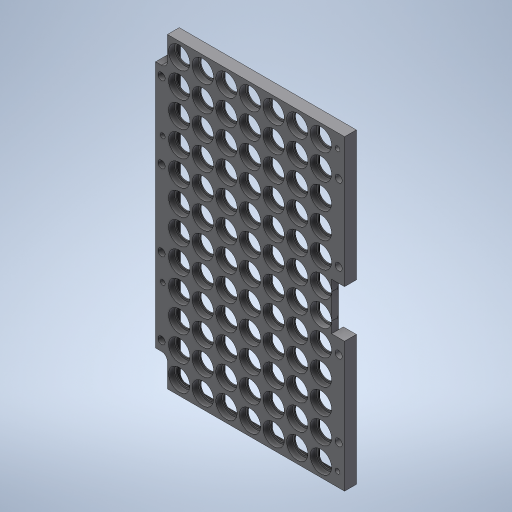
# Autodesk Inventor part: Platte2
Saved by Autodesk Inventor 2024 (Build 280153000, 153)
## iProperties
Created: 2025-03-19
Part Number: Platte2
Material: Generisch
Document SubType Name: Modeling
Designer: David Lill
Density: 1 g/cm^3
Appearance: Vorgabe
Author: David Lill
Autodesk Inventor part; units mm, degrees
ref_plane "YZ Plane" through (0, 0, 0) normal (1, 0, 0) x (0, 1, 0)
ref_plane "XZ Plane" through (0, 0, 0) normal (0, 1, 0) x (-1, 0, 0)
ref_plane "XY Plane" through (0, 0, 0) normal (0, 0, 1) x (1, 0, 0)
sketch "Skizze1" plane through (0, 0, 0) normal (0, 1, 0) x (-1, 0, 0)
  line L0 (160, 0) -> (0, 0)
  line L1 (0, 0) -> (0, -260)
  line L2 (0, -260) -> (160, -260)
  line L3 (160, -260) -> (160, 0)
  circle A0 centre (140, -11.75) radius 9
  circle A1 centre (140, -54.75) radius 9
  circle A2 centre (140, -97.75) radius 9
  circle A3 centre (140, -140.75) radius 9
  circle A4 centre (140, -183.75) radius 9
  circle A5 centre (140, -226.75) radius 9
  circle A6 centre (120, -11.75) radius 9
  circle A7 centre (120, -54.75) radius 9
  circle A8 centre (120, -97.75) radius 9
  circle A9 centre (120, -140.75) radius 9
  circle A10 centre (120, -183.75) radius 9
  circle A11 centre (120, -226.75) radius 9
  circle A12 centre (100, -11.75) radius 9
  circle A13 centre (100, -54.75) radius 9
  circle A14 centre (100, -97.75) radius 9
  circle A15 centre (100, -140.75) radius 9
  circle A16 centre (100, -183.75) radius 9
  circle A17 centre (100, -226.75) radius 9
  circle A18 centre (80, -11.75) radius 9
  circle A19 centre (80, -54.75) radius 9
  circle A20 centre (80, -97.75) radius 9
  circle A21 centre (80, -140.75) radius 9
  circle A22 centre (80, -183.75) radius 9
  circle A23 centre (80, -226.75) radius 9
  circle A24 centre (60, -11.75) radius 9
  circle A25 centre (60, -54.75) radius 9
  circle A26 centre (60, -97.75) radius 9
  circle A27 centre (60, -140.75) radius 9
  circle A28 centre (60, -183.75) radius 9
  circle A29 centre (60, -226.75) radius 9
  circle A30 centre (40, -11.75) radius 9
  circle A31 centre (40, -54.75) radius 9
  circle A32 centre (40, -97.75) radius 9
  circle A33 centre (40, -140.75) radius 9
  circle A34 centre (40, -183.75) radius 9
  circle A35 centre (40, -226.75) radius 9
  circle A36 centre (20, -11.75) radius 9
  circle A37 centre (20, -54.75) radius 9
  circle A38 centre (20, -97.75) radius 9
  circle A39 centre (20, -140.75) radius 9
  circle A40 centre (20, -183.75) radius 9
  circle A41 centre (20, -226.75) radius 9
  circle A42 centre (140, -33.25) radius 9
  circle A43 centre (120, -33.25) radius 9
  circle A44 centre (100, -33.25) radius 9
  circle A45 centre (80, -33.25) radius 9
  circle A46 centre (60, -33.25) radius 9
  circle A47 centre (40, -33.25) radius 9
  circle A48 centre (20, -33.25) radius 9
  circle A49 centre (140, -76.25) radius 9
  circle A50 centre (120, -76.25) radius 9
  circle A51 centre (100, -76.25) radius 9
  circle A52 centre (80, -76.25) radius 9
  circle A53 centre (60, -76.25) radius 9
  circle A54 centre (40, -76.25) radius 9
  circle A55 centre (20, -76.25) radius 9
  circle A56 centre (140, -119.25) radius 9
  circle A57 centre (120, -119.25) radius 9
  circle A58 centre (100, -119.25) radius 9
  circle A59 centre (80, -119.25) radius 9
  circle A60 centre (60, -119.25) radius 9
  circle A61 centre (40, -119.25) radius 9
  circle A62 centre (20, -119.25) radius 9
  circle A63 centre (140, -162.25) radius 9
  circle A64 centre (120, -162.25) radius 9
  circle A65 centre (100, -162.25) radius 9
  circle A66 centre (80, -162.25) radius 9
  circle A67 centre (60, -162.25) radius 9
  circle A68 centre (40, -162.25) radius 9
  circle A69 centre (20, -162.25) radius 9
  circle A70 centre (140, -205.25) radius 9
  circle A71 centre (120, -205.25) radius 9
  circle A72 centre (100, -205.25) radius 9
  circle A73 centre (80, -205.25) radius 9
  circle A74 centre (60, -205.25) radius 9
  circle A75 centre (40, -205.25) radius 9
  circle A76 centre (20, -205.25) radius 9
  circle A77 centre (140, -248.25) radius 9
  circle A78 centre (120, -248.25) radius 9
  circle A79 centre (100, -248.25) radius 9
  circle A80 centre (80, -248.25) radius 9
  circle A81 centre (60, -248.25) radius 9
  circle A82 centre (40, -248.25) radius 9
  circle A83 centre (20, -248.25) radius 9
  line L4 (-20, 0) -> (-187, 0)
  line L5 (-207, 0) -> (-374, 0)
  circle A84 centre (140, -11.75) radius 7.5
  line L6 (155.379, -44.5989) -> (146.379, -44.5989)
  line L7 (157, -62) -> (150, -62)
  line L8 (150, -62) -> (150, -69)
  line L9 (150, -69) -> (157, -69)
  line L10 (157, -69) -> (157, -62)
  line L11 (160, -130) -> (0, -130) construction
  line L12 (157, -198) -> (150, -198)
  line L13 (150, -198) -> (150, -191)
  line L14 (150, -191) -> (157, -191)
  line L15 (157, -191) -> (157, -198)
  point P0 (80, 0)
  point P1 (153.5, -62)
  point P2 (157, -65.5)
  dimension "d0" = 160
  dimension "d1" = 260
  dimension "d4" = 18
  dimension "d7" = 43
  dimension "d10" = 20
  dimension "d16" = 21.5
  dimension "d21" = 20
  dimension "d24" = 43
  dimension "d69" = 15
  dimension "d80" = 0
  dimension "d127" = 10.75
  dimension "d129" = 7
  dimension "d130" = 7
  dimension "d132" = 3
  dimension "d134" = 10.75
  constraints: 85 centre point, 32 end point, 14 coincident, 6 horizontal, 5 midpoint, 4 parallel, 4 symmetric about line, 2 horizontal alignment, 2 perpendicular, 2 vertical, 1 equal radius, 1 vertical alignment, 164 other
  measures "d0" distance of L0.start L0.end
  measures "d1" distance of L2.end L0.start
  measures "d4" diameter of A0
  measures "d7" distance of A0.centre A1.centre
  measures "d10" distance of A0.centre A6.centre
  measures "d16" distance of A42.centre A0.centre
  measures "d21" distance of A42.centre A43.centre
  measures "d24" distance of A42.centre A49.centre
  measures "d69" diameter of A84
  measures "d80" horizontal distance of A0.centre A42.centre
  measures "d127" vertical distance of L11.start point (140, -119.25)
  measures "d129" distance of L9.end L8.end
  measures "d130" distance of L8.end L7.end
  measures "d132" distance between parallel lines of L3 L10
  measures "d134" vertical distance of point (140, -76.25) point (157, -65.5)
extrude "Extrusion1" add sketch "Skizze1" along normal blind 10 contours L3 L2 L1 L0 | A0 | A1 | A2 | A3 | A4 | A5 | A6 | A7 | A8 | A9 | A10 | A11 | A12 | A13 | A14 | A15 | A16 | A17 | A18 | A19 | A20 | A21 | A22 | A23 | A24 | A25 | A26 | A27 | A28 | A29 | A30 | A31 | A32 | A33 | A34 | A35 | A36 | A37 | A38 | A39 | A40 | A41 | A42 | A43 | A44 | A45 | A46 | A47 | A48 | A49 | A50 | A51 | A52 | A53 | A54 | A55 | A56 | A57 | A58 | A59 | A60 | A61 | A62 | A63 | A64 | A65 | A66 | A67 | A68 | A69 | A70 | A71 | A72 | A73 | A74 | A75 | A76 | A77 | A78 | A79 | A80 | A81 | A82 | A83 | A84 | L10 L9 L8 L7 | L12 L13 L14 L15
hole "Bohrung1" at (-140, 0, -11.75) at (-140, 0, -33.25) at (-140, 0, -54.75) at (-140, 0, -76.25) at (-140, 0, -97.75) at (-140, 0, -119.25) at (-140, 0, -140.75) at (-140, 0, -162.25) at (-140, 0, -183.75) at (-140, 0, -205.25) at (-140, 0, -226.75) at (-140, 0, -248.25) direction (0, 1, 0) diameter 15 end through all counterbore diameter 18 counterbore depth 5
pattern_linear "Rechteckige Anordnung1" count 7 spacing 20 along (1, 0, 0) of "Bohrung1"
sketch "Skizze2" plane through (0, 10, 0) normal (0, 1, 0) x (1, 0, 0)
  circle A0 centre (-20, 226.75) radius 9 projected
  circle A1 centre (-20, 248.25) radius 9 projected
  circle A2 centre (-20, 205.25) radius 9 projected
  circle A3 centre (-20, 162.25) radius 9 projected
  circle A4 centre (-20, 119.25) radius 9 projected
  circle A5 centre (-20, 33.25) radius 9 projected
  circle A6 centre (-20, 11.75) radius 9
  circle A7 centre (-20, 54.75) radius 9 projected
  circle A8 centre (-20, 97.75) radius 9 projected
  circle A9 centre (-20, 140.75) radius 9 projected
  circle A10 centre (-20, 183.75) radius 9 projected
  circle A11 centre (-40, 226.75) radius 9 projected
  circle A12 centre (-40, 248.25) radius 9 projected
  circle A13 centre (-40, 205.25) radius 9 projected
  circle A14 centre (-40, 162.25) radius 9 projected
  circle A15 centre (-40, 119.25) radius 9 projected
  circle A16 centre (-40, 76.25) radius 9 projected
  circle A17 centre (-40, 33.25) radius 9 projected
  circle A18 centre (-40, 11.75) radius 9 projected
  circle A19 centre (-40, 54.75) radius 9 projected
  circle A20 centre (-40, 97.75) radius 9 projected
  circle A21 centre (-40, 140.75) radius 9 projected
  circle A22 centre (-40, 183.75) radius 9 projected
  circle A23 centre (-60, 226.75) radius 9 projected
  circle A24 centre (-60, 248.25) radius 9 projected
  circle A25 centre (-60, 205.25) radius 9 projected
  circle A26 centre (-60, 162.25) radius 9 projected
  circle A27 centre (-60, 119.25) radius 9 projected
  circle A28 centre (-60, 76.25) radius 9 projected
  circle A29 centre (-60, 33.25) radius 9 projected
  circle A30 centre (-60, 11.75) radius 9 projected
  circle A31 centre (-60, 54.75) radius 9 projected
  circle A32 centre (-60, 97.75) radius 9 projected
  circle A33 centre (-60, 140.75) radius 9 projected
  circle A34 centre (-60, 183.75) radius 9 projected
  circle A35 centre (-80, 226.75) radius 9 projected
  circle A36 centre (-80, 248.25) radius 9 projected
  circle A37 centre (-80, 205.25) radius 9 projected
  circle A38 centre (-80, 162.25) radius 9 projected
  circle A39 centre (-80, 119.25) radius 9 projected
  circle A40 centre (-80, 76.25) radius 9 projected
  circle A41 centre (-80, 33.25) radius 9 projected
  circle A42 centre (-80, 11.75) radius 9 projected
  circle A43 centre (-80, 54.75) radius 9 projected
  circle A44 centre (-80, 97.75) radius 9 projected
  circle A45 centre (-80, 140.75) radius 9 projected
  circle A46 centre (-80, 183.75) radius 9 projected
  circle A47 centre (-100, 226.75) radius 9 projected
  circle A48 centre (-100, 248.25) radius 9 projected
  circle A49 centre (-100, 205.25) radius 9 projected
  circle A50 centre (-100, 162.25) radius 9 projected
  circle A51 centre (-100, 119.25) radius 9 projected
  circle A52 centre (-100, 76.25) radius 9 projected
  circle A53 centre (-100, 33.25) radius 9 projected
  circle A54 centre (-100, 11.75) radius 9 projected
  circle A55 centre (-100, 54.75) radius 9 projected
  circle A56 centre (-100, 97.75) radius 9 projected
  circle A57 centre (-100, 140.75) radius 9 projected
  circle A58 centre (-100, 183.75) radius 9 projected
  circle A59 centre (-120, 226.75) radius 9 projected
  circle A60 centre (-120, 248.25) radius 9 projected
  circle A61 centre (-120, 205.25) radius 9 projected
  circle A62 centre (-120, 162.25) radius 9 projected
  circle A63 centre (-120, 119.25) radius 9 projected
  circle A64 centre (-120, 76.25) radius 9 projected
  circle A65 centre (-120, 33.25) radius 9 projected
  circle A66 centre (-120, 11.75) radius 9 projected
  circle A67 centre (-120, 54.75) radius 9 projected
  circle A68 centre (-120, 97.75) radius 9 projected
  circle A69 centre (-120, 140.75) radius 9 projected
  circle A70 centre (-120, 183.75) radius 9 projected
  circle A71 centre (-140, 226.75) radius 9 projected
  circle A72 centre (-140, 183.75) radius 9 projected
  circle A73 centre (-140, 140.75) radius 9 projected
  circle A74 centre (-140, 97.75) radius 9 projected
  circle A75 centre (-140, 54.75) radius 9 projected
  circle A76 centre (-140, 11.75) radius 9 projected
  circle A77 centre (-140, 33.25) radius 9 projected
  circle A78 centre (-140, 76.25) radius 9 projected
  circle A79 centre (-140, 119.25) radius 9 projected
  circle A80 centre (-140, 162.25) radius 9 projected
  circle A81 centre (-140, 205.25) radius 9 projected
  circle A82 centre (-140, 248.25) radius 9 projected
  line L0 (0, 0) -> (0, 260) projected
  line L1 (-160, 0) -> (0, 0) projected
  line L2 (-160, 260) -> (-160, 0) projected
  line L3 (0, 260) -> (-160, 260) projected
  line L4 (-160, 0) -> (0, 0) projected
  line L5 (-150, 0) -> (-150, 55)
  arc A83 (-150, 55) -> (-155, 60) centre (-155, 55) ccw
  line L6 (-155, 60) -> (-160, 60)
  line L7 (-160, 260) -> (-160, 0) projected
  line L8 (-160, 0) -> (0, 0) projected
  line L9 (0, 0) -> (0, 260) projected
  line L10 (-160, 260) -> (-160, 0) projected
  line L11 (0, 260) -> (-160, 260) projected
  line L12 (-160, 25) -> (-155, 25)
  arc A84 (-150, 20) -> (-155, 25) centre (-155, 20) ccw
  line L13 (0, 130) -> (-160, 130)
  line L14 (-150, 260) -> (-150, 205)
  arc A85 (-155, 200) -> (-150, 205) centre (-155, 205) ccw
  line L15 (-155, 200) -> (-160, 200)
  line L16 (-160, 235) -> (-155, 235)
  arc A86 (-155, 235) -> (-150, 240) centre (-155, 240) ccw
  circle A87 centre (-20, 11.75) radius 9 projected
  line L17 (-143.0414, 85.25) -> (-151, 85.25)
  arc A88 (-151, 85.25) -> (-151, 67.25) centre (-151, 76.25) ccw
  line L18 (-151, 67.25) -> (-143.0414, 67.25)
  arc A89 (-143.0414, 85.25) -> (-143.0414, 67.25) centre (-140, 76.25) ccw
  line L19 (-143.0414, 174.75) -> (-151, 174.75)
  arc A90 (-151, 192.75) -> (-151, 174.75) centre (-151, 183.75) ccw
  line L20 (-151, 192.75) -> (-143.0414, 192.75)
  arc A91 (-143.0414, 192.75) -> (-143.0414, 174.75) centre (-140, 183.75) ccw
  circle A92 centre (-154, 76.25) radius 4
  circle A93 centre (-154, 183.75) radius 4
  line L21 (-80, 260) -> (-80, 0)
  line L22 (0, 232.75) -> (-3, 232.75)
  arc A94 (-3, 232.75) -> (-3, 220.75) centre (-3, 226.75) ccw
  line L23 (-3, 220.75) -> (0, 220.75)
  line L24 (0, 168.25) -> (-3, 168.25)
  arc A95 (-3, 168.25) -> (-3, 156.25) centre (-3, 162.25) ccw
  line L25 (-3, 156.25) -> (0, 156.25)
  line L26 (-160, 168.25) -> (-157, 168.25)
  arc A96 (-157, 156.25) -> (-157, 168.25) centre (-157, 162.25) ccw
  line L27 (-157, 156.25) -> (-160, 156.25)
  line L28 (0, 27.25) -> (-3, 27.25)
  arc A97 (-3, 39.25) -> (-3, 27.25) centre (-3, 33.25) ccw
  line L29 (-3, 39.25) -> (0, 39.25)
  line L30 (0, 91.75) -> (-3, 91.75)
  arc A98 (-3, 103.75) -> (-3, 91.75) centre (-3, 97.75) ccw
  line L31 (-3, 103.75) -> (0, 103.75)
  arc A99 (-157, 91.75) -> (-157, 103.75) centre (-157, 97.75) ccw
  line L32 (-160, 91.75) -> (-157, 91.75)
  line L33 (-157, 103.75) -> (-160, 103.75)
  line L34 (-16.9586, 20.75) -> (-9, 20.75)
  arc A100 (-9, 2.75) -> (-9, 20.75) centre (-9, 11.75) ccw
  line L35 (-9, 2.75) -> (-16.9586, 2.75)
  arc A101 (-16.9586, 2.75) -> (-16.9586, 20.75) centre (-20, 11.75) ccw
  circle A102 centre (-6, 11.75) radius 4
  arc A103 (-9, 239.25) -> (-9, 257.25) centre (-9, 248.25) ccw
  line L36 (-9, 257.25) -> (-16.9586, 257.25)
  arc A104 (-16.9586, 239.25) -> (-16.9586, 257.25) centre (-20, 248.25) ccw
  line L37 (-16.9586, 239.25) -> (-9, 239.25)
  circle A105 centre (-6, 248.25) radius 4
  line L38 (-160, 232.75) -> (-157, 232.75)
  arc A106 (-157, 220.75) -> (-157, 232.75) centre (-157, 226.75) ccw
  line L39 (-157, 220.75) -> (-160, 220.75)
  arc A107 (-157, 27.25) -> (-157, 39.25) centre (-157, 33.25) ccw
  line L40 (-160, 27.25) -> (-157, 27.25)
  line L41 (-157, 39.25) -> (-160, 39.25)
  line L42 (-11, 199.5) -> (-3, 199.5)
  line L43 (-3, 199.5) -> (-3, 179.5)
  line L44 (-3, 179.5) -> (-11, 179.5)
  line L45 (-11, 179.5) -> (-11, 199.5)
  line L46 (-11, 60.5) -> (-3, 60.5)
  line L47 (-3, 60.5) -> (-3, 80.5)
  line L48 (-3, 80.5) -> (-11, 80.5)
  line L49 (-11, 80.5) -> (-11, 60.5)
  line L50 (-156.36, 69) -> (-149.36, 69)
  line L51 (-149.36, 69) -> (-149.36, 62)
  line L52 (-149.36, 62) -> (-156.36, 62)
  line L53 (-156.36, 62) -> (-156.36, 69)
  line L54 (-156.36, 191) -> (-149.36, 191)
  line L55 (-149.36, 191) -> (-149.36, 198)
  line L56 (-149.36, 198) -> (-156.36, 198)
  line L57 (-156.36, 198) -> (-156.36, 191)
  point P0 (-160, 60)
  point P1 (0, 130)
  point P2 (-150, 260)
  point P3 (-160, 200)
  point P4 (-160, 235)
  point P5 (-160, 25)
  point P6 (0, 27.25)
  point P7 (0, 39.25)
  point P8 (0, 103.75)
  point P9 (-5, 226.75)
  point P10 (-5, 162.25)
  point P11 (-5, 33.25)
  point P12 (-5, 97.75)
  point P13 (-155, 226.75)
  point P14 (-155, 162.25)
  point P15 (-155, 97.75)
  point P16 (-155, 33.25)
  point P17 (-7, 199.5)
  point P18 (-7, 179.5)
  point P19 (-3, 189.5)
  point P20 (-11, 189.5)
  point P21 (-152.86, 69)
  point P22 (-149.36, 65.5)
  dimension "d83" = 10
  dimension "d84" = 5
  dimension "d85" = 60
  dimension "d101" = 25
  dimension "d119" = 8
  dimension "d121" = 6
  dimension "d124" = 33.25
  dimension "d125" = 64.5
  dimension "d126" = 6
  dimension "d135" = 9.5
  dimension "d136" = 3
  dimension "d142" = 6
  dimension "d143" = 5
  dimension "d144" = 5
  dimension "d160" = 8
  dimension "d162" = 3
  dimension "d165" = 20
  dimension "d166" = 5.75
  dimension "d169" = 7
  dimension "d170" = 7
  dimension "d171" = 3.64
  dimension "d172" = 10.75
  constraints: 107 centre point, 96 end point, 68 symmetric about line, 40 point on circle, 14 tangent, 11 midpoint, 9 point on line, 7 horizontal, 7 parallel, 7 perpendicular, 6 coincident, 6 equal radius, 6 horizontal alignment, 2 vertical, 2 vertical alignment, 1 concentric, 14 other
  measures "d83" distance between parallel lines of L2 L5
  measures "d84" radius of A83
  measures "d85" distance between parallel lines of L6 L4
  measures "d101" distance between parallel lines of L4 L12
  measures "d119" diameter of A92
  measures "d121" distance from line of L2 A92.centre
  measures "d124" distance from line of L11 point (-3, 226.75)
  measures "d125" distance of point (-3, 226.75) point (-3, 162.25)
  measures "d126" radius of A94
  measures "d135" radius of A89
  measures "d136" distance from line of L0 point (-3, 226.75)
  measures "d142" distance from line of L9 A102.centre
  measures "d143" distance from line of L0 point (-5, 226.75)
  measures "d144" distance from line of L0 point (-5, 162.25)
  measures "d160" distance of point (-3, 189.5) point (-11, 189.5)
  measures "d162" distance from line of L9 L42.end
  measures "d165" distance of L42.end L43.end
  measures "d166" distance from line of A2.centre L42
  measures "d169" distance from line of L52 point (-152.86, 69)
  measures "d170" distance of L50.start L50.end
  measures "d171" distance between parallel lines of L10 L53
  measures "d172" vertical distance of A89.centre point (-149.36, 65.5)
extrude "Extrusion2" cut sketch "Skizze2" against normal blind 10 contours L14 A86 L16 L2 L3 | L12 A84 L5 L1 L2
sketch "Skizze3" plane through (0, 10, 0) normal (0, 1, 0) x (1, 0, 0)
  point P0 (0, 0)
sketch "Skizze4" plane through (0, 10, 0) normal (0, 1, 0) x (1, 0, 0)
  line L0 (-150, 0) -> (0, 0) projected
  line L1 (0, 260) -> (-150, 260) projected
  line L2 (-16, 258) -> (-144, 258)
  line L3 (-144, 2) -> (-16, 2)
  arc A0 (-16, 2) -> (-11, 7) centre (-16, 7) ccw
  line L4 (-11, 7) -> (-11, 253)
  arc A1 (-11, 253) -> (-16, 258) centre (-16, 253) ccw
  circle A2 centre (-20, 248.25) radius 7.5 projected
  arc A3 (-149, 7) -> (-144, 2) centre (-144, 7) ccw
  arc A4 (-144, 258) -> (-149, 253) centre (-144, 253) ccw
  line L5 (-149, 253) -> (-149, 7)
  circle A5 centre (-140, 248.25) radius 7.5 projected
  arc A6 (-3, 103.75) -> (-3, 91.75) centre (-3, 97.75) ccw projected
  line L6 (-3, 103.75) -> (0, 103.75) projected
  line L7 (0, 91.75) -> (-3, 91.75) projected
  line L8 (0, 0) -> (0, 260) projected
  line L9 (0, 0) -> (0, 260) projected
  line L10 (0, 156.25) -> (-3, 156.25) projected
  arc A7 (-3, 168.25) -> (-3, 156.25) centre (-3, 162.25) ccw projected
  line L11 (-3, 168.25) -> (0, 168.25) projected
  line L12 (0, 0) -> (0, 260) projected
  line L13 (0, 0) -> (0, 260) projected
  line L14 (-3, 232.75) -> (0, 232.75) projected
  arc A8 (-3, 232.75) -> (-3, 220.75) centre (-3, 226.75) ccw projected
  line L15 (0, 220.75) -> (-3, 220.75) projected
  line L16 (0, 0) -> (0, 260) projected
  line L17 (-3, 39.25) -> (0, 39.25) projected
  arc A9 (-3, 39.25) -> (-3, 27.25) centre (-3, 33.25) ccw projected
  line L18 (0, 27.25) -> (-3, 27.25) projected
  line L19 (-150, 260) -> (-150, 240) projected
  arc A10 (-155, 235) -> (-150, 240) centre (-155, 240) ccw projected
  line L20 (-155, 235) -> (-160, 235) projected
  arc A11 (-157, 220.75) -> (-157, 232.75) centre (-157, 226.75) ccw projected
  line L21 (-160, 235) -> (-160, 25) projected
  line L22 (-157, 220.75) -> (-160, 220.75) projected
  line L23 (-160, 232.75) -> (-157, 232.75) projected
  line L24 (-160, 235) -> (-160, 25) projected
  line L25 (-157, 156.25) -> (-160, 156.25) projected
  arc A12 (-157, 156.25) -> (-157, 168.25) centre (-157, 162.25) ccw projected
  line L26 (-160, 168.25) -> (-157, 168.25) projected
  line L27 (-160, 235) -> (-160, 25) projected
  line L28 (-160, 103.75) -> (-157, 103.75) projected
  arc A13 (-157, 91.75) -> (-157, 103.75) centre (-157, 97.75) ccw projected
  line L29 (-157, 91.75) -> (-160, 91.75) projected
  line L30 (-160, 235) -> (-160, 25) projected
  line L31 (-150, 20) -> (-150, 0) projected
  arc A14 (-150, 20) -> (-155, 25) centre (-155, 20) ccw projected
  line L32 (-160, 25) -> (-155, 25) projected
  line L33 (-160, 235) -> (-160, 25) projected
  line L34 (-157, 27.25) -> (-160, 27.25) projected
  arc A15 (-157, 27.25) -> (-157, 39.25) centre (-157, 33.25) ccw projected
  line L35 (-160, 39.25) -> (-157, 39.25) projected
  circle A16 centre (-6, 11.75) radius 3 projected
  circle A17 centre (-6, 248.25) radius 3 projected
  circle A18 centre (-154, 76.25) radius 3 projected
  circle A19 centre (-154, 183.75) radius 3 projected
  line L36 (-11, 110) -> (0, 110)
  line L37 (-11, 150) -> (0, 150)
  line L38 (-144, 2) -> (-150, 2)
  line L39 (-144, 258) -> (-150, 258)
  arc A20 (-154, 62) -> (-149, 67) centre (-154, 67) ccw
  line L40 (-154, 62) -> (-160, 62)
  line L41 (-160, 198) -> (-154, 198)
  arc A21 (-149, 193) -> (-154, 198) centre (-154, 193) ccw
  point P0 (-154.75, 102.7936)
  point P1 (-154.75, 157.2064)
  point P2 (-154.75, 38.2936)
  point P3 (-154.75, 73.3453)
  point P4 (-154.75, 79.1547)
  point P5 (-154.75, 92.7064)
  point P6 (-150, 20)
  point P7 (-154.75, 28.2064)
  point P8 (-154.75, 231.7936)
  point P9 (-154.75, 167.2936)
  point P10 (-154.75, 180.8453)
  point P11 (-154.75, 186.6547)
  point P12 (-154.75, 221.7064)
  point P13 (-150, 252)
  point P14 (-5.25, 251.1547)
  point P15 (-3, 248.25)
  point P16 (-3, 232.6661)
  point P17 (-3, 220.8339)
  point P18 (-3, 168.1661)
  point P19 (-3, 156.3339)
  point P20 (-3, 103.6661)
  point P21 (-3, 91.8339)
  point P22 (-3, 39.1661)
  point P23 (-3, 27.3339)
  point P24 (-3, 11.75)
  point P25 (-5.25, 8.8453)
  point P26 (-150, 8)
  point P27 (-11, 130)
  point P28 (0, 33.25)
  point P29 (-160, 162.25)
  point P30 (0, 33.25)
  point P31 (0, 39.25)
  point P32 (-160, 162.25)
  dimension "d180" = 2
  dimension "d181" = 2
  dimension "d182" = 5
  dimension "d184" = 9
  dimension "d185" = 9
  dimension "d190" = 40
  dimension "d191" = 20
  dimension "d195" = 60
  dimension "d196" = 60
  constraints: 20 end point, 12 point on circle, 12 tangent, 10 point on line, 6 centre point, 5 equal radius, 4 perpendicular, 2 horizontal, 2 parallel, 2 vertical, 1 midpoint
  measures "d180" distance between parallel lines of L1 L2
  measures "d181" distance between parallel lines of L0 L3
  measures "d182" radius of A1
  measures "d184" distance from line of L5 A5.centre
  measures "d185" distance from line of A2.centre L4
  measures "d190" distance between parallel lines of L37 L36
  measures "d191" distance from line of point (-11, 130) L36
  measures "d195" distance between parallel lines of L40 L38
  measures "d196" distance between parallel lines of L41 L39
extrude "Extrusion6" cut sketch "Skizze4" against normal blind 4 contours A3 L5 A4 L2 A1 L4 A0 L3
extrude "Extrusion7" cut sketch "Skizze4" along normal through all both and the other way through all contours L4 L37 L8 L36
sketch "Skizze5" plane through (0, 0, 0) normal (0, -1, 0) x (1, 0, 0)
  point P0 (0, 0)
  point P1 (-5, -33.25)
  point P2 (-5, -97.75)
  point P3 (-5, -162.25)
  point P4 (-5, -226.75)
  point P5 (-155, -226.75)
  point P6 (-155, -162.25)
  point P7 (-155, -97.75)
  point P8 (-155, -33.25)
hole "Bohrung5" at (-5, 0, -33.25) at (-5, 0, -97.75) at (-5, 0, -162.25) at (-5, 0, -226.75) at (-155, 0, -226.75) at (-155, 0, -162.25) at (-155, 0, -97.75) at (-155, 0, -33.25) direction (0, 1, 0) diameter 4 end through all counterbore diameter 6 counterbore depth 5
hole "Bohrung6" at (-6, 10, -11.75) at (-6, 10, -248.25) at (-154, 10, -183.75) at (-154, 10, -76.25) direction (0, -1, 0) diameter 4 end through all counterbore diameter 6 counterbore depth 5
sketch "Skizze6" plane through (0, 6, 0) normal (0, 1, 0) x (1, 0, 0)
  line L0 (-149, 7) -> (-149, 253) projected
  arc A0 (-116.25, 131) -> (-111.25, 136) centre (-116.25, 136) ccw
  line L1 (-111.25, 136) -> (-111.25, 253)
  arc A1 (-111.25, 253) -> (-116.25, 258) centre (-116.25, 253) ccw
  line L2 (-116.25, 258) -> (-144, 258)
  arc A2 (-144, 258) -> (-149, 253) centre (-144, 253) ccw
  line L3 (-149, 253) -> (-149, 136)
  arc A3 (-149, 136) -> (-144, 131) centre (-144, 136) ccw
  line L4 (-144, 131) -> (-116.25, 131)
  line L5 (-145.125, 243.25) -> (-145.125, 253.25)
  line L6 (-145.125, 253.25) -> (-135.125, 253.25)
  line L7 (-135.125, 253.25) -> (-135.125, 243.25)
  line L8 (-135.125, 243.25) -> (-145.125, 243.25)
  line L9 (-125.125, 243.25) -> (-125.125, 253.25)
  line L10 (-125.125, 253.25) -> (-115.125, 253.25)
  line L11 (-115.125, 253.25) -> (-115.125, 243.25)
  line L12 (-115.125, 243.25) -> (-125.125, 243.25)
  line L13 (-145.125, 221.75) -> (-145.125, 231.75)
  line L14 (-145.125, 231.75) -> (-135.125, 231.75)
  line L15 (-135.125, 231.75) -> (-135.125, 221.75)
  line L16 (-135.125, 221.75) -> (-145.125, 221.75)
  line L17 (-125.125, 221.75) -> (-125.125, 231.75)
  line L18 (-125.125, 231.75) -> (-115.125, 231.75)
  line L19 (-115.125, 231.75) -> (-115.125, 221.75)
  line L20 (-115.125, 221.75) -> (-125.125, 221.75)
  line L21 (-145.125, 200.25) -> (-145.125, 210.25)
  line L22 (-145.125, 210.25) -> (-135.125, 210.25)
  line L23 (-135.125, 210.25) -> (-135.125, 200.25)
  line L24 (-135.125, 200.25) -> (-145.125, 200.25)
  line L25 (-125.125, 200.25) -> (-125.125, 210.25)
  line L26 (-125.125, 210.25) -> (-115.125, 210.25)
  line L27 (-115.125, 210.25) -> (-115.125, 200.25)
  line L28 (-115.125, 200.25) -> (-125.125, 200.25)
  line L29 (-145.125, 178.75) -> (-145.125, 188.75)
  line L30 (-145.125, 188.75) -> (-135.125, 188.75)
  line L31 (-135.125, 188.75) -> (-135.125, 178.75)
  line L32 (-135.125, 178.75) -> (-145.125, 178.75)
  line L33 (-125.125, 178.75) -> (-125.125, 188.75)
  line L34 (-125.125, 188.75) -> (-115.125, 188.75)
  line L35 (-115.125, 188.75) -> (-115.125, 178.75)
  line L36 (-115.125, 178.75) -> (-125.125, 178.75)
  line L37 (-145.125, 157.25) -> (-145.125, 167.25)
  line L38 (-145.125, 167.25) -> (-135.125, 167.25)
  line L39 (-135.125, 167.25) -> (-135.125, 157.25)
  line L40 (-135.125, 157.25) -> (-145.125, 157.25)
  line L41 (-125.125, 157.25) -> (-125.125, 167.25)
  line L42 (-125.125, 167.25) -> (-115.125, 167.25)
  line L43 (-115.125, 167.25) -> (-115.125, 157.25)
  line L44 (-115.125, 157.25) -> (-125.125, 157.25)
  line L45 (-145.125, 135.75) -> (-145.125, 145.75)
  line L46 (-145.125, 145.75) -> (-135.125, 145.75)
  line L47 (-135.125, 145.75) -> (-135.125, 135.75)
  line L48 (-135.125, 135.75) -> (-145.125, 135.75)
  line L49 (-115.125, 135.75) -> (-125.125, 135.75)
  line L50 (-125.125, 135.75) -> (-125.125, 145.75)
  line L51 (-125.125, 145.75) -> (-115.125, 145.75)
  line L52 (-115.125, 145.75) -> (-115.125, 135.75)
  line L53 (-109, 253) -> (-109, 136)
  line L54 (-105.125, 178.75) -> (-105.125, 188.75)
  line L55 (-95.125, 178.75) -> (-105.125, 178.75)
  line L56 (-105.125, 188.75) -> (-95.125, 188.75)
  line L57 (-95.125, 188.75) -> (-95.125, 178.75)
  line L58 (-85.125, 178.75) -> (-85.125, 188.75)
  line L59 (-85.125, 200.25) -> (-85.125, 210.25)
  line L60 (-75.125, 178.75) -> (-85.125, 178.75)
  line L61 (-75.125, 200.25) -> (-85.125, 200.25)
  line L62 (-75.125, 188.75) -> (-75.125, 178.75)
  line L63 (-85.125, 188.75) -> (-75.125, 188.75)
  line L64 (-75.125, 210.25) -> (-75.125, 200.25)
  line L65 (-85.125, 210.25) -> (-75.125, 210.25)
  line L66 (-71.25, 136) -> (-71.25, 253)
  line L67 (-95.125, 210.25) -> (-95.125, 200.25)
  line L68 (-95.125, 200.25) -> (-105.125, 200.25)
  line L69 (-105.125, 200.25) -> (-105.125, 210.25)
  line L70 (-105.125, 210.25) -> (-95.125, 210.25)
  line L71 (-95.125, 221.75) -> (-105.125, 221.75)
  line L72 (-95.125, 231.75) -> (-95.125, 221.75)
  line L73 (-105.125, 231.75) -> (-95.125, 231.75)
  line L74 (-105.125, 221.75) -> (-105.125, 231.75)
  line L75 (-75.125, 221.75) -> (-85.125, 221.75)
  line L76 (-85.125, 221.75) -> (-85.125, 231.75)
  line L77 (-75.125, 231.75) -> (-75.125, 221.75)
  line L78 (-85.125, 231.75) -> (-75.125, 231.75)
  line L79 (-75.125, 243.25) -> (-85.125, 243.25)
  line L80 (-85.125, 253.25) -> (-75.125, 253.25)
  line L81 (-75.125, 253.25) -> (-75.125, 243.25)
  line L82 (-85.125, 243.25) -> (-85.125, 253.25)
  line L83 (-95.125, 243.25) -> (-105.125, 243.25)
  arc A4 (-71.25, 253) -> (-76.25, 258) centre (-76.25, 253) ccw
  line L84 (-95.125, 253.25) -> (-95.125, 243.25)
  line L85 (-105.125, 243.25) -> (-105.125, 253.25)
  line L86 (-105.125, 253.25) -> (-95.125, 253.25)
  arc A5 (-104, 258) -> (-109, 253) centre (-104, 253) ccw
  line L87 (-76.25, 258) -> (-104, 258)
  line L88 (-85.125, 167.25) -> (-75.125, 167.25)
  line L89 (-105.125, 167.25) -> (-95.125, 167.25)
  line L90 (-105.125, 157.25) -> (-105.125, 167.25)
  line L91 (-95.125, 167.25) -> (-95.125, 157.25)
  line L92 (-85.125, 157.25) -> (-85.125, 167.25)
  line L93 (-95.125, 157.25) -> (-105.125, 157.25)
  line L94 (-75.125, 157.25) -> (-85.125, 157.25)
  line L95 (-85.125, 145.75) -> (-75.125, 145.75)
  line L96 (-105.125, 145.75) -> (-95.125, 145.75)
  line L97 (-75.125, 145.75) -> (-75.125, 135.75)
  line L98 (-75.125, 135.75) -> (-85.125, 135.75)
  line L99 (-85.125, 135.75) -> (-85.125, 145.75)
  line L100 (-95.125, 145.75) -> (-95.125, 135.75)
  line L101 (-105.125, 135.75) -> (-105.125, 145.75)
  line L102 (-95.125, 135.75) -> (-105.125, 135.75)
  arc A6 (-109, 136) -> (-104, 131) centre (-104, 136) ccw
  line L103 (-104, 131) -> (-76.25, 131)
  arc A7 (-76.25, 131) -> (-71.25, 136) centre (-76.25, 136) ccw
  line L104 (-75.125, 167.25) -> (-75.125, 157.25)
  line L105 (-69, 253) -> (-69, 136)
  line L106 (-65.125, 178.75) -> (-65.125, 188.75)
  line L107 (-55.125, 178.75) -> (-65.125, 178.75)
  line L108 (-65.125, 188.75) -> (-55.125, 188.75)
  line L109 (-55.125, 188.75) -> (-55.125, 178.75)
  line L110 (-45.125, 178.75) -> (-45.125, 188.75)
  line L111 (-45.125, 200.25) -> (-45.125, 210.25)
  line L112 (-35.125, 178.75) -> (-45.125, 178.75)
  line L113 (-35.125, 200.25) -> (-45.125, 200.25)
  line L114 (-35.125, 188.75) -> (-35.125, 178.75)
  line L115 (-45.125, 188.75) -> (-35.125, 188.75)
  line L116 (-35.125, 210.25) -> (-35.125, 200.25)
  line L117 (-45.125, 210.25) -> (-35.125, 210.25)
  line L118 (-31.25, 136) -> (-31.25, 253)
  line L119 (-55.125, 210.25) -> (-55.125, 200.25)
  line L120 (-55.125, 200.25) -> (-65.125, 200.25)
  line L121 (-65.125, 200.25) -> (-65.125, 210.25)
  line L122 (-65.125, 210.25) -> (-55.125, 210.25)
  line L123 (-55.125, 221.75) -> (-65.125, 221.75)
  line L124 (-55.125, 231.75) -> (-55.125, 221.75)
  line L125 (-65.125, 231.75) -> (-55.125, 231.75)
  line L126 (-65.125, 221.75) -> (-65.125, 231.75)
  line L127 (-35.125, 221.75) -> (-45.125, 221.75)
  line L128 (-45.125, 221.75) -> (-45.125, 231.75)
  line L129 (-35.125, 231.75) -> (-35.125, 221.75)
  line L130 (-45.125, 231.75) -> (-35.125, 231.75)
  line L131 (-35.125, 243.25) -> (-45.125, 243.25)
  line L132 (-45.125, 253.25) -> (-35.125, 253.25)
  line L133 (-35.125, 253.25) -> (-35.125, 243.25)
  line L134 (-45.125, 243.25) -> (-45.125, 253.25)
  line L135 (-55.125, 243.25) -> (-65.125, 243.25)
  arc A8 (-31.25, 253) -> (-36.25, 258) centre (-36.25, 253) ccw
  line L136 (-55.125, 253.25) -> (-55.125, 243.25)
  line L137 (-65.125, 243.25) -> (-65.125, 253.25)
  line L138 (-65.125, 253.25) -> (-55.125, 253.25)
  arc A9 (-64, 258) -> (-69, 253) centre (-64, 253) ccw
  line L139 (-36.25, 258) -> (-64, 258)
  line L140 (-45.125, 167.25) -> (-35.125, 167.25)
  line L141 (-65.125, 167.25) -> (-55.125, 167.25)
  line L142 (-65.125, 157.25) -> (-65.125, 167.25)
  line L143 (-55.125, 167.25) -> (-55.125, 157.25)
  line L144 (-45.125, 157.25) -> (-45.125, 167.25)
  line L145 (-55.125, 157.25) -> (-65.125, 157.25)
  line L146 (-35.125, 157.25) -> (-45.125, 157.25)
  line L147 (-45.125, 145.75) -> (-35.125, 145.75)
  line L148 (-65.125, 145.75) -> (-55.125, 145.75)
  line L149 (-35.125, 145.75) -> (-35.125, 135.75)
  line L150 (-35.125, 135.75) -> (-45.125, 135.75)
  line L151 (-45.125, 135.75) -> (-45.125, 145.75)
  line L152 (-55.125, 145.75) -> (-55.125, 135.75)
  line L153 (-65.125, 135.75) -> (-65.125, 145.75)
  line L154 (-55.125, 135.75) -> (-65.125, 135.75)
  arc A10 (-69, 136) -> (-64, 131) centre (-64, 136) ccw
  line L155 (-64, 131) -> (-36.25, 131)
  arc A11 (-36.25, 131) -> (-31.25, 136) centre (-36.25, 136) ccw
  line L156 (-35.125, 167.25) -> (-35.125, 157.25)
  line L157 (-149, 124) -> (-149, 7)
  line L158 (-145.125, 49.75) -> (-145.125, 59.75)
  line L159 (-135.125, 49.75) -> (-145.125, 49.75)
  line L160 (-145.125, 59.75) -> (-135.125, 59.75)
  line L161 (-135.125, 59.75) -> (-135.125, 49.75)
  line L162 (-125.125, 49.75) -> (-125.125, 59.75)
  line L163 (-125.125, 71.25) -> (-125.125, 81.25)
  line L164 (-115.125, 49.75) -> (-125.125, 49.75)
  line L165 (-115.125, 71.25) -> (-125.125, 71.25)
  line L166 (-115.125, 59.75) -> (-115.125, 49.75)
  line L167 (-125.125, 59.75) -> (-115.125, 59.75)
  line L168 (-115.125, 81.25) -> (-115.125, 71.25)
  line L169 (-125.125, 81.25) -> (-115.125, 81.25)
  line L170 (-111.25, 7) -> (-111.25, 124)
  line L171 (-135.125, 81.25) -> (-135.125, 71.25)
  line L172 (-135.125, 71.25) -> (-145.125, 71.25)
  line L173 (-145.125, 71.25) -> (-145.125, 81.25)
  line L174 (-145.125, 81.25) -> (-135.125, 81.25)
  line L175 (-135.125, 92.75) -> (-145.125, 92.75)
  line L176 (-135.125, 102.75) -> (-135.125, 92.75)
  line L177 (-145.125, 102.75) -> (-135.125, 102.75)
  line L178 (-145.125, 92.75) -> (-145.125, 102.75)
  line L179 (-115.125, 92.75) -> (-125.125, 92.75)
  line L180 (-125.125, 92.75) -> (-125.125, 102.75)
  line L181 (-115.125, 102.75) -> (-115.125, 92.75)
  line L182 (-125.125, 102.75) -> (-115.125, 102.75)
  line L183 (-115.125, 114.25) -> (-125.125, 114.25)
  line L184 (-125.125, 124.25) -> (-115.125, 124.25)
  line L185 (-115.125, 124.25) -> (-115.125, 114.25)
  line L186 (-125.125, 114.25) -> (-125.125, 124.25)
  line L187 (-135.125, 114.25) -> (-145.125, 114.25)
  arc A12 (-111.25, 124) -> (-116.25, 129) centre (-116.25, 124) ccw
  line L188 (-135.125, 124.25) -> (-135.125, 114.25)
  line L189 (-145.125, 114.25) -> (-145.125, 124.25)
  line L190 (-145.125, 124.25) -> (-135.125, 124.25)
  arc A13 (-144, 129) -> (-149, 124) centre (-144, 124) ccw
  line L191 (-116.25, 129) -> (-144, 129)
  line L192 (-125.125, 38.25) -> (-115.125, 38.25)
  line L193 (-145.125, 38.25) -> (-135.125, 38.25)
  line L194 (-145.125, 28.25) -> (-145.125, 38.25)
  line L195 (-135.125, 38.25) -> (-135.125, 28.25)
  line L196 (-125.125, 28.25) -> (-125.125, 38.25)
  line L197 (-135.125, 28.25) -> (-145.125, 28.25)
  line L198 (-115.125, 28.25) -> (-125.125, 28.25)
  line L199 (-125.125, 16.75) -> (-115.125, 16.75)
  line L200 (-145.125, 16.75) -> (-135.125, 16.75)
  line L201 (-115.125, 16.75) -> (-115.125, 6.75)
  line L202 (-115.125, 6.75) -> (-125.125, 6.75)
  line L203 (-125.125, 6.75) -> (-125.125, 16.75)
  line L204 (-135.125, 16.75) -> (-135.125, 6.75)
  line L205 (-145.125, 6.75) -> (-145.125, 16.75)
  line L206 (-135.125, 6.75) -> (-145.125, 6.75)
  arc A14 (-149, 7) -> (-144, 2) centre (-144, 7) ccw
  line L207 (-144, 2) -> (-116.25, 2)
  arc A15 (-116.25, 2) -> (-111.25, 7) centre (-116.25, 7) ccw
  line L208 (-115.125, 38.25) -> (-115.125, 28.25)
  line L209 (-109, 124) -> (-109, 7)
  line L210 (-105.125, 49.75) -> (-105.125, 59.75)
  line L211 (-95.125, 49.75) -> (-105.125, 49.75)
  line L212 (-105.125, 59.75) -> (-95.125, 59.75)
  line L213 (-95.125, 59.75) -> (-95.125, 49.75)
  line L214 (-85.125, 49.75) -> (-85.125, 59.75)
  line L215 (-85.125, 71.25) -> (-85.125, 81.25)
  line L216 (-75.125, 49.75) -> (-85.125, 49.75)
  line L217 (-75.125, 71.25) -> (-85.125, 71.25)
  line L218 (-75.125, 59.75) -> (-75.125, 49.75)
  line L219 (-85.125, 59.75) -> (-75.125, 59.75)
  line L220 (-75.125, 81.25) -> (-75.125, 71.25)
  line L221 (-85.125, 81.25) -> (-75.125, 81.25)
  line L222 (-71.25, 7) -> (-71.25, 124)
  line L223 (-95.125, 81.25) -> (-95.125, 71.25)
  line L224 (-95.125, 71.25) -> (-105.125, 71.25)
  line L225 (-105.125, 71.25) -> (-105.125, 81.25)
  line L226 (-105.125, 81.25) -> (-95.125, 81.25)
  line L227 (-95.125, 92.75) -> (-105.125, 92.75)
  line L228 (-95.125, 102.75) -> (-95.125, 92.75)
  line L229 (-105.125, 102.75) -> (-95.125, 102.75)
  line L230 (-105.125, 92.75) -> (-105.125, 102.75)
  line L231 (-75.125, 92.75) -> (-85.125, 92.75)
  line L232 (-85.125, 92.75) -> (-85.125, 102.75)
  line L233 (-75.125, 102.75) -> (-75.125, 92.75)
  line L234 (-85.125, 102.75) -> (-75.125, 102.75)
  line L235 (-75.125, 114.25) -> (-85.125, 114.25)
  line L236 (-85.125, 124.25) -> (-75.125, 124.25)
  line L237 (-75.125, 124.25) -> (-75.125, 114.25)
  line L238 (-85.125, 114.25) -> (-85.125, 124.25)
  line L239 (-95.125, 114.25) -> (-105.125, 114.25)
  arc A16 (-71.25, 124) -> (-76.25, 129) centre (-76.25, 124) ccw
  line L240 (-95.125, 124.25) -> (-95.125, 114.25)
  line L241 (-105.125, 114.25) -> (-105.125, 124.25)
  line L242 (-105.125, 124.25) -> (-95.125, 124.25)
  arc A17 (-104, 129) -> (-109, 124) centre (-104, 124) ccw
  line L243 (-76.25, 129) -> (-104, 129)
  line L244 (-85.125, 38.25) -> (-75.125, 38.25)
  line L245 (-105.125, 38.25) -> (-95.125, 38.25)
  line L246 (-105.125, 28.25) -> (-105.125, 38.25)
  line L247 (-95.125, 38.25) -> (-95.125, 28.25)
  line L248 (-85.125, 28.25) -> (-85.125, 38.25)
  line L249 (-95.125, 28.25) -> (-105.125, 28.25)
  line L250 (-75.125, 28.25) -> (-85.125, 28.25)
  line L251 (-85.125, 16.75) -> (-75.125, 16.75)
  line L252 (-105.125, 16.75) -> (-95.125, 16.75)
  line L253 (-75.125, 16.75) -> (-75.125, 6.75)
  line L254 (-75.125, 6.75) -> (-85.125, 6.75)
  line L255 (-85.125, 6.75) -> (-85.125, 16.75)
  line L256 (-95.125, 16.75) -> (-95.125, 6.75)
  line L257 (-105.125, 6.75) -> (-105.125, 16.75)
  line L258 (-95.125, 6.75) -> (-105.125, 6.75)
  arc A18 (-109, 7) -> (-104, 2) centre (-104, 7) ccw
  line L259 (-104, 2) -> (-76.25, 2)
  arc A19 (-76.25, 2) -> (-71.25, 7) centre (-76.25, 7) ccw
  line L260 (-75.125, 38.25) -> (-75.125, 28.25)
  line L261 (-69, 124) -> (-69, 7)
  line L262 (-65.125, 49.75) -> (-65.125, 59.75)
  line L263 (-55.125, 49.75) -> (-65.125, 49.75)
  line L264 (-65.125, 59.75) -> (-55.125, 59.75)
  line L265 (-55.125, 59.75) -> (-55.125, 49.75)
  line L266 (-45.125, 49.75) -> (-45.125, 59.75)
  line L267 (-45.125, 71.25) -> (-45.125, 81.25)
  line L268 (-35.125, 49.75) -> (-45.125, 49.75)
  line L269 (-35.125, 71.25) -> (-45.125, 71.25)
  line L270 (-35.125, 59.75) -> (-35.125, 49.75)
  line L271 (-45.125, 59.75) -> (-35.125, 59.75)
  line L272 (-35.125, 81.25) -> (-35.125, 71.25)
  line L273 (-45.125, 81.25) -> (-35.125, 81.25)
  line L274 (-31.25, 7) -> (-31.25, 124)
  line L275 (-55.125, 81.25) -> (-55.125, 71.25)
  line L276 (-55.125, 71.25) -> (-65.125, 71.25)
  line L277 (-65.125, 71.25) -> (-65.125, 81.25)
  line L278 (-65.125, 81.25) -> (-55.125, 81.25)
  line L279 (-55.125, 92.75) -> (-65.125, 92.75)
  line L280 (-55.125, 102.75) -> (-55.125, 92.75)
  line L281 (-65.125, 102.75) -> (-55.125, 102.75)
  line L282 (-65.125, 92.75) -> (-65.125, 102.75)
  line L283 (-35.125, 92.75) -> (-45.125, 92.75)
  line L284 (-45.125, 92.75) -> (-45.125, 102.75)
  line L285 (-35.125, 102.75) -> (-35.125, 92.75)
  line L286 (-45.125, 102.75) -> (-35.125, 102.75)
  line L287 (-35.125, 114.25) -> (-45.125, 114.25)
  line L288 (-45.125, 124.25) -> (-35.125, 124.25)
  line L289 (-35.125, 124.25) -> (-35.125, 114.25)
  line L290 (-45.125, 114.25) -> (-45.125, 124.25)
  line L291 (-55.125, 114.25) -> (-65.125, 114.25)
  arc A20 (-31.25, 124) -> (-36.25, 129) centre (-36.25, 124) ccw
  line L292 (-55.125, 124.25) -> (-55.125, 114.25)
  line L293 (-65.125, 114.25) -> (-65.125, 124.25)
  line L294 (-65.125, 124.25) -> (-55.125, 124.25)
  arc A21 (-64, 129) -> (-69, 124) centre (-64, 124) ccw
  line L295 (-36.25, 129) -> (-64, 129)
  line L296 (-45.125, 38.25) -> (-35.125, 38.25)
  line L297 (-65.125, 38.25) -> (-55.125, 38.25)
  line L298 (-65.125, 28.25) -> (-65.125, 38.25)
  line L299 (-55.125, 38.25) -> (-55.125, 28.25)
  line L300 (-45.125, 28.25) -> (-45.125, 38.25)
  line L301 (-55.125, 28.25) -> (-65.125, 28.25)
  line L302 (-35.125, 28.25) -> (-45.125, 28.25)
  line L303 (-45.125, 16.75) -> (-35.125, 16.75)
  line L304 (-65.125, 16.75) -> (-55.125, 16.75)
  line L305 (-35.125, 16.75) -> (-35.125, 6.75)
  line L306 (-35.125, 6.75) -> (-45.125, 6.75)
  line L307 (-45.125, 6.75) -> (-45.125, 16.75)
  line L308 (-55.125, 16.75) -> (-55.125, 6.75)
  line L309 (-65.125, 6.75) -> (-65.125, 16.75)
  line L310 (-55.125, 6.75) -> (-65.125, 6.75)
  arc A22 (-69, 7) -> (-64, 2) centre (-64, 7) ccw
  line L311 (-64, 2) -> (-36.25, 2)
  arc A23 (-36.25, 2) -> (-31.25, 7) centre (-36.25, 7) ccw
  line L312 (-35.125, 38.25) -> (-35.125, 28.25)
  circle A24 centre (-20, 226.75) radius 7.5 projected
  circle A25 centre (-20, 205.25) radius 7.5 projected
  circle A26 centre (-20, 162.25) radius 7.5 projected
  circle A27 centre (-20, 119.25) radius 7.5 projected
  circle A28 centre (-20, 76.25) radius 7.5 projected
  circle A29 centre (-20, 33.25) radius 7.5 projected
  circle A30 centre (-20, 11.75) radius 7.5 projected
  circle A31 centre (-20, 54.75) radius 7.5 projected
  circle A32 centre (-20, 97.75) radius 7.5 projected
  circle A33 centre (-20, 140.75) radius 7.5 projected
  circle A34 centre (-20, 183.75) radius 7.5 projected
  circle A35 centre (-40, 226.75) radius 7.5 projected
  circle A36 centre (-40, 248.25) radius 7.5 projected
  circle A37 centre (-40, 205.25) radius 7.5 projected
  circle A38 centre (-40, 162.25) radius 7.5 projected
  circle A39 centre (-40, 119.25) radius 7.5 projected
  circle A40 centre (-40, 76.25) radius 7.5 projected
  circle A41 centre (-40, 33.25) radius 7.5 projected
  circle A42 centre (-40, 11.75) radius 7.5 projected
  circle A43 centre (-40, 54.75) radius 7.5 projected
  circle A44 centre (-40, 97.75) radius 7.5 projected
  circle A45 centre (-40, 140.75) radius 7.5 projected
  circle A46 centre (-40, 183.75) radius 7.5 projected
  circle A47 centre (-60, 226.75) radius 7.5 projected
  circle A48 centre (-60, 248.25) radius 7.5 projected
  circle A49 centre (-60, 205.25) radius 7.5 projected
  circle A50 centre (-60, 162.25) radius 7.5 projected
  circle A51 centre (-60, 119.25) radius 7.5 projected
  circle A52 centre (-60, 76.25) radius 7.5 projected
  circle A53 centre (-60, 33.25) radius 7.5 projected
  circle A54 centre (-60, 11.75) radius 7.5 projected
  circle A55 centre (-60, 54.75) radius 7.5 projected
  circle A56 centre (-60, 97.75) radius 7.5 projected
  circle A57 centre (-60, 140.75) radius 7.5 projected
  circle A58 centre (-60, 183.75) radius 7.5 projected
  circle A59 centre (-80, 226.75) radius 7.5 projected
  circle A60 centre (-80, 248.25) radius 7.5 projected
  circle A61 centre (-80, 205.25) radius 7.5 projected
  circle A62 centre (-80, 162.25) radius 7.5 projected
  circle A63 centre (-80, 119.25) radius 7.5 projected
  circle A64 centre (-80, 76.25) radius 7.5 projected
  circle A65 centre (-80, 33.25) radius 7.5 projected
  circle A66 centre (-80, 11.75) radius 7.5 projected
  circle A67 centre (-80, 54.75) radius 7.5 projected
  circle A68 centre (-80, 97.75) radius 7.5 projected
  circle A69 centre (-80, 140.75) radius 7.5 projected
  circle A70 centre (-80, 183.75) radius 7.5 projected
  circle A71 centre (-100, 226.75) radius 7.5 projected
  circle A72 centre (-100, 248.25) radius 7.5 projected
  circle A73 centre (-100, 205.25) radius 7.5 projected
  circle A74 centre (-100, 162.25) radius 7.5 projected
  circle A75 centre (-100, 119.25) radius 7.5 projected
  circle A76 centre (-100, 76.25) radius 7.5 projected
  circle A77 centre (-100, 33.25) radius 7.5 projected
  circle A78 centre (-100, 11.75) radius 7.5 projected
  circle A79 centre (-100, 54.75) radius 7.5 projected
  circle A80 centre (-100, 97.75) radius 7.5 projected
  circle A81 centre (-100, 140.75) radius 7.5 projected
  circle A82 centre (-100, 183.75) radius 7.5 projected
  circle A83 centre (-120, 226.75) radius 7.5 projected
  circle A84 centre (-120, 248.25) radius 7.5 projected
  circle A85 centre (-120, 205.25) radius 7.5 projected
  circle A86 centre (-120, 162.25) radius 7.5 projected
  circle A87 centre (-120, 119.25) radius 7.5 projected
  circle A88 centre (-120, 76.25) radius 7.5 projected
  circle A89 centre (-120, 33.25) radius 7.5 projected
  circle A90 centre (-120, 11.75) radius 7.5 projected
  circle A91 centre (-120, 54.75) radius 7.5 projected
  circle A92 centre (-120, 97.75) radius 7.5 projected
  circle A93 centre (-120, 140.75) radius 7.5 projected
  circle A94 centre (-120, 183.75) radius 7.5 projected
  circle A95 centre (-140, 226.75) radius 7.5 projected
  circle A96 centre (-140, 183.75) radius 7.5 projected
  circle A97 centre (-140, 140.75) radius 7.5 projected
  circle A98 centre (-140, 97.75) radius 7.5 projected
  circle A99 centre (-140, 54.75) radius 7.5 projected
  circle A100 centre (-140, 11.75) radius 7.5 projected
  circle A101 centre (-140, 33.25) radius 7.5 projected
  circle A102 centre (-140, 76.25) radius 7.5 projected
  circle A103 centre (-140, 119.25) radius 7.5 projected
  circle A104 centre (-140, 162.25) radius 7.5 projected
  circle A105 centre (-140, 205.25) radius 7.5 projected
  line L313 (-149, 7) -> (-149, 253) projected
  arc A106 (-149, 7) -> (-144, 2) centre (-144, 7) ccw projected
  line L314 (-16, 2) -> (-144, 2) projected
  arc A107 (-16, 2) -> (-11, 7) centre (-16, 7) ccw projected
  line L315 (-11, 110) -> (-11, 7) projected
  line L316 (-11, 150) -> (-11, 110) projected
  line L317 (-11, 253) -> (-11, 150) projected
  arc A108 (-11, 253) -> (-16, 258) centre (-16, 253) ccw projected
  line L318 (-144, 258) -> (-16, 258) projected
  arc A109 (-144, 258) -> (-149, 253) centre (-144, 253) ccw projected
  circle A110 centre (-140, 248.25) radius 7.5 projected
  circle A111 centre (-20, 248.25) radius 7.5 projected
  arc A112 (-11, 253) -> (-16, 258) centre (-16, 253) ccw projected
  arc A113 (-24, 258) -> (-29, 253) centre (-24, 253) ccw
  line L319 (-29, 253) -> (-29, 7)
  arc A114 (-29, 7) -> (-24, 2) centre (-24, 7) ccw
  line L320 (-24, 2) -> (-16, 2)
  arc A115 (-16, 2) -> (-11, 7) centre (-16, 7) ccw
  line L321 (-11, 7) -> (-11, 253)
  arc A116 (-11, 253) -> (-16, 258) centre (-16, 253) ccw
  line L322 (-16, 258) -> (-24, 258)
  line L323 (-25.25, 6.75) -> (-25.25, 16.75)
  line L324 (-25.25, 16.75) -> (-15.25, 16.75)
  line L325 (-15.25, 16.75) -> (-15.25, 6.75)
  line L326 (-15.25, 6.75) -> (-25.25, 6.75)
  line L327 (-25.25, 28.25) -> (-25.25, 38.25)
  line L328 (-25.25, 38.25) -> (-15.25, 38.25)
  line L329 (-15.25, 38.25) -> (-15.25, 28.25)
  line L330 (-15.25, 28.25) -> (-25.25, 28.25)
  line L331 (-25.25, 49.75) -> (-25.25, 59.75)
  line L332 (-25.25, 59.75) -> (-15.25, 59.75)
  line L333 (-15.25, 59.75) -> (-15.25, 49.75)
  line L334 (-15.25, 49.75) -> (-25.25, 49.75)
  line L335 (-25.25, 71.25) -> (-25.25, 81.25)
  line L336 (-25.25, 81.25) -> (-15.25, 81.25)
  line L337 (-15.25, 81.25) -> (-15.25, 71.25)
  line L338 (-15.25, 71.25) -> (-25.25, 71.25)
  line L339 (-25.25, 92.75) -> (-25.25, 102.75)
  line L340 (-25.25, 102.75) -> (-15.25, 102.75)
  line L341 (-15.25, 102.75) -> (-15.25, 92.75)
  line L342 (-15.25, 92.75) -> (-25.25, 92.75)
  line L343 (-25.25, 114.25) -> (-25.25, 124.25)
  line L344 (-25.25, 124.25) -> (-15.25, 124.25)
  line L345 (-15.25, 124.25) -> (-15.25, 114.25)
  line L346 (-15.25, 114.25) -> (-25.25, 114.25)
  line L347 (-25.25, 135.75) -> (-25.25, 145.75)
  line L348 (-25.25, 145.75) -> (-15.25, 145.75)
  line L349 (-15.25, 145.75) -> (-15.25, 135.75)
  line L350 (-15.25, 135.75) -> (-25.25, 135.75)
  line L351 (-25.25, 157.25) -> (-25.25, 167.25)
  line L352 (-25.25, 167.25) -> (-15.25, 167.25)
  line L353 (-15.25, 167.25) -> (-15.25, 157.25)
  line L354 (-15.25, 157.25) -> (-25.25, 157.25)
  line L355 (-25.25, 178.75) -> (-25.25, 188.75)
  line L356 (-25.25, 188.75) -> (-15.25, 188.75)
  line L357 (-15.25, 188.75) -> (-15.25, 178.75)
  line L358 (-15.25, 178.75) -> (-25.25, 178.75)
  line L359 (-25.25, 200.25) -> (-25.25, 210.25)
  line L360 (-25.25, 210.25) -> (-15.25, 210.25)
  line L361 (-15.25, 210.25) -> (-15.25, 200.25)
  line L362 (-15.25, 200.25) -> (-25.25, 200.25)
  line L363 (-25.25, 221.75) -> (-25.25, 231.75)
  line L364 (-25.25, 231.75) -> (-15.25, 231.75)
  line L365 (-15.25, 231.75) -> (-15.25, 221.75)
  line L366 (-15.25, 221.75) -> (-25.25, 221.75)
  line L367 (-25.25, 253.25) -> (-15.25, 253.25)
  line L368 (-15.25, 253.25) -> (-15.25, 243.25)
  line L369 (-15.25, 243.25) -> (-25.25, 243.25)
  line L370 (-25.25, 243.25) -> (-25.25, 253.25)
  point P0 (0, 0)
  point P1 (-111.25, 131)
  point P2 (-71.25, 131)
  point P3 (-31.25, 131)
  point P4 (-111.25, 2)
  point P5 (-71.25, 2)
  point P6 (-31.25, 2)
  point P7 (-29, 258)
  point P8 (-104, 2)
  point P9 (-64, 2)
  point P10 (-24, 2)
  dimension "d213" = 40
  dimension "d216" = 129
  constraints: 728 end point, 56 point on circle, 56 vertical, 55 horizontal, 28 centre point, 1 collinear, 756 other
  measures "d213" distance of L0.end point (-109, 253)
  measures "d216" distance of L0.end point (-149, 124)
extrude "Extrusion8" add sketch "Skizze6" along normal blind 2 contours L0 A3 L4 A0 L1 A1 L318 A5 L53 A6 L103 A7 L66 A4 A9 L105 A10 L155 A11 L118 A8 A113 L319 A114 L314 A23 L274 A20 L295 A21 L261 A22 A19 L222 A16 L243 A17 L209 A18 A15 L170 A12 L191 A13
equation "\"d16\" = 0.5 * d7"
equation "\"d21\" = d10"
equation "\"d24\" = d7"
